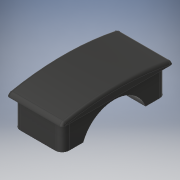
# Autodesk Inventor part: ARM_087_IntakeSideCap(WithCutout)
Saved by Autodesk Inventor 2018 (Build 220112000, 112)
## iProperties
Created: 2020-02-12
Part Number: ARM_087_IntakeSideCap(WithCutout)
Material: ABS Plastic
Document SubType Name: Modeling
Designer: Team20
Density: 1.06 g/cm^3
Appearance: Smooth - White
Mass: 12.7734 g
Surface Area: 42.7754 cm^2
Volume: 12.0504 cm^3
Author: Team20
Autodesk Inventor part; units mm, degrees
ref_plane "YZ Plane" through (0, 0, 0) normal (1, 0, 0) x (0, 1, 0)
ref_plane "XZ Plane" through (0, 0, 0) normal (0, 1, 0) x (-1, 0, 0)
ref_plane "XY Plane" through (0, 0, 0) normal (0, 0, 1) x (1, 0, 0)
sketch "Sketch1" plane through (0, 0, 0) normal (0, 1, 0) x (-1, 0, 0)
  line L0 (-7.9375, 23.8125) -> (7.9375, 23.8125)
  line L1 (11.1125, 20.6375) -> (11.1125, -20.6375)
  line L2 (7.9375, -23.8125) -> (-7.9375, -23.8125)
  line L3 (-11.1125, -20.6375) -> (-11.1125, 20.6375)
  line L4 (-11.1125, 23.8125) -> (11.1125, -23.8125) construction
  line L5 (11.1125, 23.8125) -> (-11.1125, -23.8125) construction
  arc A0 (7.9375, -23.8125) -> (11.1125, -20.6375) centre (7.9375, -20.6375) ccw
  arc A1 (-11.1125, -20.6375) -> (-7.9375, -23.8125) centre (-7.9375, -20.6375) ccw
  arc A2 (-7.9375, 23.8125) -> (-11.1125, 20.6375) centre (-7.9375, 20.6375) ccw
  arc A3 (11.1125, 20.6375) -> (7.9375, 23.8125) centre (7.9375, 20.6375) ccw
  point P0 (0, 0)
  dimension "d0" = 47.625
  dimension "d1" = 22.225
  dimension "d15" = 3.175
  constraints: 12 end point, 8 point on circle, 8 point on line, 8 tangent, 4 centre point, 3 equal radius, 2 midpoint, 2 parallel, 1 horizontal, 1 perpendicular
  measures "d0" distance of L5.start L4.end
  measures "d1" distance of L4.start L5.start
  measures "d15" radius of A0
extrude "Extrusion1" add sketch "Sketch1" along normal mid plane 12.065
sketch "Sketch3" plane through (0, -6.0325, -23.8125) normal (1, 0, 0) x (0, 0, -1)
  line L0 (-44.45, 12.065) -> (-3.175, 12.065) projected
  line L1 (-3.175, 0) -> (-44.45, 0) projected
  line L2 (-49.2125, 12.065) -> (1.5875, 12.065)
  arc A0 (-47.625, 13.6525) -> (-49.2125, 12.065) centre (-47.2211, 11.6611) ccw
  arc A1 (1.5875, 12.065) -> (0, 13.6525) centre (-0.4039, 11.6611) ccw
  arc A2 (0, 13.6525) -> (-47.625, 13.6525) centre (-23.8125, -103.7429) ccw
  line L3 (-3.175, 12.065) -> (-3.175, 0) projected
  line L4 (-44.45, 12.065) -> (-44.45, 0) projected
  point P0 (-23.8125, 6.0325)
  point P1 (-47.625, 12.065)
  dimension "d5" = 50.8
  dimension "d9" = 1.5875
  dimension "d13" = 2.032
  dimension "d14" = 2.032
  constraints: 6 point on circle, 3 centre point, 2 end point, 1 collinear, 1 horizontal, 1 point on line, 1 tangent
  measures "d5" distance of L2.start L2.end
  measures "d9" distance of point (-47.625, 12.065) A0.start
  measures "d13" radius of A0
  measures "d14" radius of A1
extrude "Extrusion2" add sketch "Sketch3" along normal mid plane 25.4 contours L2 A0 A2 A1 L0
fillet "Fillet1" radius 1.27 6 edges at (-12.7, 7.0654, -24.8454) (-12.7, 7.0654, 24.8454) (-12.7, 10.0107, 0) (12.7, 7.0654, 24.8454) (12.7, 7.0654, -24.8454) (12.7, 10.0107, 0)
sketch "Sketch4" plane through (11.1125, -6.0325, 20.6375) normal (1, 0, 0) x (0, 0, -1)
  line L0 (41.275, 12.065) -> (0, 12.065) projected
  line L1 (20.6375, 12.065) -> (20.6375, -5.4102)
  circle A0 centre (20.6375, -5.4102) radius 15.24
  point P0 (20.6375, 6.0325)
  dimension "d17" = 17.4752
  dimension "d18" = 30.48
  constraints: 2 end point, 1 centre point, 1 coincident, 1 midpoint, 1 vertical
  measures "d17" distance of L1.start L1.end
  measures "d18" diameter of A0
extrude "Extrusion3" cut sketch "Sketch4" against normal blind 127
body "Solid1"
